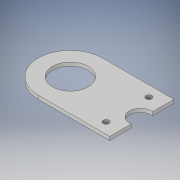
# Autodesk Inventor part: motor extension
Saved by Autodesk Inventor 2019 (Build 230136000, 136)
## iProperties
Created: 2019-01-19
Part Number: motor extension
Material: Generic
Document SubType Name: Modeling
Designer: Tiberus
Density: 1 g/cm^3
Appearance: Default
Author: Tiberus
Autodesk Inventor part; units mm, degrees
ref_plane "YZ Plane" through (0, 0, 0) normal (1, 0, 0) x (0, 1, 0)
ref_plane "XZ Plane" through (0, 0, 0) normal (0, 1, 0) x (-1, 0, 0)
ref_plane "XY Plane" through (0, 0, 0) normal (0, 0, 1) x (1, 0, 0)
sketch "Sketch1" plane through (0, 0, 0) normal (0, 1, 0) x (-1, 0, 0)
  circle A0 centre (0, 0) radius 15.875
  arc A1 (0, -28.575) -> (0, 28.575) centre (0, 0) ccw
  line L0 (0, 28.575) -> (-63.5, 28.575)
  line L1 (-63.5, -28.575) -> (0, -28.575)
  line L2 (-36.1351, 28.575) -> (-36.1351, 9.525) construction
  line L3 (-36.1351, -28.575) -> (-36.1351, -9.525) construction
  line L4 (-63.5, 28.575) -> (-63.5, 9.525)
  line L5 (-63.5, -9.525) -> (-63.5, -28.575)
  line L6 (-63.5, 19.05) -> (-50.8, 19.05) construction
  line L7 (-63.5, -19.05) -> (-50.8, -19.05) construction
  arc A2 (-63.5, -9.525) -> (-63.5, 9.525) centre (-62.2343, 0) ccw
  circle A3 centre (-50.8, 19.05) radius 2.5797
  circle A4 centre (-50.8, -19.05) radius 2.5797
  dimension "d0" = 31.75
  dimension "d1" = 12.7
  dimension "d2" = 63.5
  dimension "d3" = 19.05
  dimension "d4" = 19.05
  dimension "d5" = 12.7
  dimension "d6" = 63.5
  dimension "d7" = 19.05
  dimension "d8" = 19.05
  dimension "d9" = 5.1594
  dimension "d10" = 5.1594
  constraints: 16 end point, 5 centre point, 4 perpendicular, 4 point on circle, 3 coincident, 3 horizontal, 2 midpoint, 2 parallel, 2 point on line, 1 tangent, 1 vertical
  measures "d0" diameter of A0
  measures "d1" radial gap between concentric circles of A0 A1
  measures "d2" distance of L0.start L0.end
  measures "d3" distance of L2.start L2.end
  measures "d4" distance of L3.start L3.end
  measures "d5" distance of L6.start L6.end
  measures "d6" distance of L1.start L1.end
  measures "d7" distance of L5.start L1.start
  measures "d8" distance of L0.end L4.end
  measures "d9" diameter of A3
  measures "d10" diameter of A4
extrude "Extrusion1" add sketch "Sketch1" along normal blind 3.175
body "Solid1"
